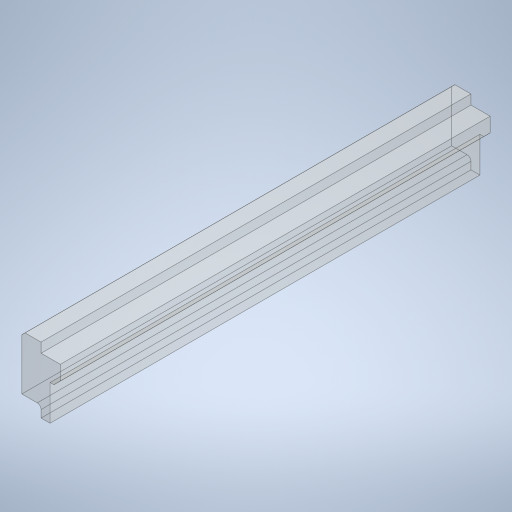
# Autodesk Inventor part: Diffuser
Saved by Autodesk Inventor 2023 (Build 270158000, 158)
## iProperties
Created: 2024-03-20
Part Number: Diffuser
Material: Glass
Document SubType Name: Modeling
Designer: noname
Density: 2.18 g/cm^3
Appearance: Clear
Author: noname
Autodesk Inventor part; units mm, degrees
ref_plane "YZ Plane" through (0, 0, 0) normal (1, 0, 0) x (0, 1, 0)
ref_plane "XZ Plane" through (0, 0, 0) normal (0, 1, 0) x (-1, 0, 0)
ref_plane "XY Plane" through (0, 0, 0) normal (0, 0, 1) x (1, 0, 0)
sketch "Sketch1" plane through (0, 0, 0) normal (0, 0, 1) x (1, 0, 0)
  line L0 (0, 12) -> (0, 9.75) construction
  line L1 (0, 0) -> (-3, 0) construction
  line L2 (-3, 0) -> (-3, 4.4) construction
  line L3 (-3.6, 5) -> (-6, 5)
  line L4 (-6, 5) -> (-6, 13)
  line L5 (-5.5, 13.5) -> (-3, 13.5)
  line L6 (-3, 13.5) -> (-3, 12)
  line L7 (-3, 12) -> (0, 12)
  line L8 (0, 3.25) -> (-1.6, 3.25) construction
  line L9 (-1.6, 3.25) -> (-1.6, 8.75)
  line L10 (-1.6, 8.75) -> (-1, 8.75)
  line L11 (0, 8.75) -> (0, 3.25)
  line L12 (0, 8.75) -> (0, 12)
  arc A0 (-3, 4.4) -> (-3.6, 5) centre (-3.6, 4.4) ccw
  line L13 (-1.6, 3.25) -> (-1.6, 0) construction
  line L14 (-3, 0) -> (-1.6, 0) construction
  line L15 (-1.6, 3.25) -> (-3, 3.25)
  line L16 (-3, 3.25) -> (-3, 4.4)
  line L17 (-1, 8.75) -> (0, 9.75)
  line L18 (-6, 13) -> (-5.5, 13.5)
  point P0 (-6, 13.5)
  point P1 (-1.6, 6)
  point P2 (0, 9.5)
  point P3 (0, 9.75)
  dimension "d0" = 12
  dimension "d1" = 3
  dimension "d2" = 3
  dimension "d3" = 5
  dimension "d4" = 1.5
  dimension "d5" = 3
  dimension "d8" = 6
  dimension "d9" = 5.5
  dimension "d14" = 1.6
  dimension "d15" = 0.6
  dimension "d16" = 1
  dimension "d17" = 1
  dimension "d18" = 0.5
  dimension "d19" = 0.5
  constraints: 38 end point, 9 point on line, 8 perpendicular, 2 collinear, 2 horizontal, 2 parallel, 2 point on circle, 2 tangent, 2 vertical, 1 centre point, 1 midpoint
  measures "d0" distance of L0.start L1.start
  measures "d1" distance between parallel lines of L0 L2
  measures "d2" distance between parallel lines of L2 L4
  measures "d3" distance between parallel lines of L1 L3
  measures "d4" distance between parallel lines of L7 L5
  measures "d5" distance between parallel lines of L0 L6
  measures "d8" distance from line of L1 point (-1.6, 6)
  measures "d9" distance between parallel lines of L8 L10
  measures "d14" distance between parallel lines of L0 L9
  measures "d15" radius of A0
  measures "d16" distance of L10.end point (0, 8.75)
  measures "d17" distance of L0.end point (0, 8.75)
  measures "d18" distance of L4.end point (-6, 13.5)
  measures "d19" distance of L5.start point (-6, 13.5)
extrude "Extrusion1" add sketch "Sketch1" along normal blind 67
body "Solid1"
